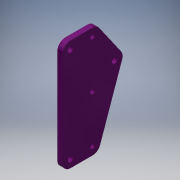
# Autodesk Inventor part: carriage plate square
Saved by Autodesk Inventor 2017 SP1 (Build 210196100, 196)
## iProperties
Created: 2018-01-19
Part Number: carriage plate square
Material: Aluminum 6061
Document SubType Name: Modeling
Designer: Ben
Density: 2.7 g/cm^3
Appearance: Smooth - Purple
Mass: 99.9601 g
Surface Area: 141.524 cm^2
Volume: 37.0222 cm^3
Author: Ben
Autodesk Inventor part; units mm, degrees
ref_plane "YZ Plane" through (0, 0, 0) normal (1, 0, 0) x (0, 1, 0)
ref_plane "XZ Plane" through (0, 0, 0) normal (0, 1, 0) x (-1, 0, 0)
ref_plane "XY Plane" through (0, 0, 0) normal (0, 0, 1) x (1, 0, 0)
sketch "Sketch1" plane through (0, 0, 0) normal (1, 0, 0) x (0, 1, 0)
  line L0 (-420.7503, 12.7) -> (420.7488, 12.7) construction
  line L1 (420.7488, 12.7) -> (420.7488, -12.7)
  line L2 (420.7488, -12.7) -> (-420.7503, -12.7) construction
  line L3 (-420.7503, -12.7) -> (-420.7503, 12.7)
  line L4 (0, 0) -> (0, -26.6192) construction
  circle A0 centre (0, -26.6192) radius 3.302
  circle A1 centre (38.1, 26.6192) radius 3.302
  circle A2 centre (-76.2, 26.6192) radius 3.302
  line L5 (38.1, 26.6192) -> (-76.2, 26.6192) construction
  line L6 (0, 0) -> (0, 26.6192) construction
  circle A3 centre (0, -26.6192) radius 15.875 construction
  circle A4 centre (38.1, 26.6192) radius 15.875 construction
  circle A5 centre (-76.2, 26.6192) radius 15.875 construction
  line L7 (0, -26.6192) -> (-76.2, 26.6192) construction
  arc A6 (47.625, 26.6192) -> (38.1, 36.1442) centre (38.1, 26.6192) ccw
  arc A7 (-76.2, 36.1442) -> (-85.725, 26.6192) centre (-76.2, 26.6192) ccw
  line L8 (38.1, 36.1442) -> (-76.2, 36.1442)
  line L9 (47.625, 26.6192) -> (47.625, 0)
  line L10 (-85.725, 0) -> (-85.725, 26.6192)
  line L11 (-76.2, 26.6192) -> (-76.2, 0) construction
  line L12 (38.1, 26.6192) -> (38.1, 0) construction
  circle A8 centre (38.1, 0) radius 2.667
  circle A9 centre (-76.2, 0) radius 2.667
  line L13 (47.625, 0) -> (-85.725, 0) construction
  line L14 (-85.725, 0) -> (-420.7503, 0) construction
  circle A10 centre (-19.05, 0) radius 2.667
  arc A11 (43.5552, -7.8081) -> (47.625, 0) centre (38.1, 0) ccw
  arc A12 (-85.725, 0) -> (-79.3412, -8.9921) centre (-76.2, 0) ccw
  arc A13 (-3.1412, -35.6113) -> (5.4552, -34.4273) centre (0, -26.6192) ccw
  line L15 (43.5552, -7.8081) -> (5.4552, -34.4273)
  line L16 (-3.1412, -35.6113) -> (-79.3412, -8.9921)
  line L17 (0, -26.6192) -> (38.1, 26.6192) construction
  dimension "d0" = 25.4
  dimension "d1" = 6.604
  dimension "d2" = 13.9192
  dimension "d3" = 31.75
  dimension "d4" = 38.1
  dimension "d5" = 76.2
  dimension "d6" = 9.525
  dimension "d9" = 5.334
  constraints: 36 end point, 14 centre point, 12 coincident, 10 point on circle, 9 tangent, 8 equal radius, 6 point on line, 5 vertical, 3 horizontal, 3 perpendicular, 2 collinear, 2 midpoint, 2 parallel
  measures "d0" distance of L0.end L1.end
  measures "d1" diameter of A0
  measures "d2" distance from line of L2 L4.end
  measures "d3" diameter of A3
  measures "d4" horizontal distance of L5.start L4.end
  measures "d5" distance from line of A2.centre L6
  measures "d6" radius of A6
  measures "d9" diameter of A8
extrude "Extrusion1" add sketch "Sketch1" along normal blind 6.35
body "Solid1"
